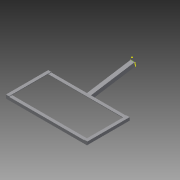
# Autodesk Inventor part: Prow rev2
Saved by Autodesk Inventor 2015 (Build 190159000, 159)
## iProperties
Created: 2016-02-01
Part Number: Prow rev2
Material: Generic
Document SubType Name: Modeling
Designer: sethbattis
Density: 1 g/cm^3
Appearance: Default
Author: sethbattis
Autodesk Inventor part; units mm, degrees
ref_plane "YZ Plane" through (0, 0, 0) normal (1, 0, 0) x (0, 1, 0)
ref_plane "XZ Plane" through (0, 0, 0) normal (0, 1, 0) x (-1, 0, 0)
ref_plane "XY Plane" through (0, 0, 0) normal (0, 0, 1) x (1, 0, 0)
sketch "Sketch1" plane through (0, 0, 0) normal (1, 0, 0) x (0, 1, 0)
  line L0 (-3.175, 114.3) -> (0, 114.3)
  line L1 (0, 114.3) -> (0, 133.35)
  line L2 (0, 133.35) -> (-19.05, 133.35)
  line L3 (-19.05, 133.35) -> (-19.05, 130.175)
  line L4 (-19.05, 130.175) -> (-3.175, 130.175)
  line L5 (-3.175, 130.175) -> (-3.175, 114.3)
  line L6 (0, -114.3) -> (0, -133.35)
  line L7 (0, -133.35) -> (-19.05, -133.35)
  line L8 (-19.05, -133.35) -> (-19.05, -130.175)
  line L9 (-19.05, -130.175) -> (-3.175, -130.175)
  line L10 (-3.175, -130.175) -> (-3.175, -114.3)
  line L11 (-3.175, -114.3) -> (0, -114.3)
  line L12 (-25.4768, 0) -> (19.5105, 0) construction
  line L13 (0, -349.8749) -> (0, 213.8875) construction
  point P0 (0, 0)
  dimension "d0" = 19.05
  dimension "d1" = 19.05
  dimension "d3" = 266.7
  dimension "d4" = 3.175
  constraints: 24 end point, 9 perpendicular, 5 equal length, 2 point on line, 1 collinear, 1 horizontal, 1 vertical, 1 other
  measures "d0" distance of L1.end L2.end
  measures "d1" distance of L0.end L1.end
  measures "d3" distance between parallel lines of L7 L2
  measures "d4" distance of L0.start L0.end
extrude "Extrusion1" add sketch "Sketch1" along normal mid plane 508
sketch "Sketch3" plane through (0, 0, 0) normal (1, 0, 0) x (0, 1, 0)
  line L0 (-25.0873, -137.3234) -> (18.6205, -413.2836)
  line L1 (0, -323.2049) -> (0, 53.8675) projected
  line L2 (-25.0873, -137.3234) -> (0, -133.35)
  line L3 (0, -133.35) -> (43.7078, -409.3101)
  line L4 (43.7078, -409.3101) -> (18.6205, -413.2836)
  point P0 (0, 0)
  dimension "d7" = 9
  dimension "d8" = 279.4
  dimension "d10" = 25.4
  constraints: 8 end point, 3 perpendicular
  measures "d7" angle of L1 L0
  measures "d8" distance of L2.end L3.end
  measures "d10" distance of L2.end L0.start
extrude "Extrusion2" add sketch "Sketch3" along normal mid plane 25.4
sketch "Sketch4" plane through (-254, -19.05, 133.35) normal (0, 0, 1) x (1, 0, 0)
  line L0 (241.3, 19.05) -> (0, 19.05) projected
  line L1 (15.875, 19.05) -> (15.875, 22.225)
  line L2 (15.875, 22.225) -> (-3.175, 22.225)
  line L3 (-3.175, 22.225) -> (-3.175, 3.175)
  line L4 (-3.175, 3.175) -> (0, 3.175)
  line L5 (0, 3.175) -> (0, 19.05)
  line L6 (0, 19.05) -> (15.875, 19.05)
  line L7 (492.028, 19.05) -> (492.028, 22.225)
  line L8 (492.028, 22.225) -> (511.078, 22.225)
  line L9 (511.078, 22.225) -> (511.078, 3.175)
  line L10 (511.078, 3.175) -> (507.903, 3.175)
  line L11 (507.903, 3.175) -> (507.903, 19.05)
  line L12 (507.903, 19.05) -> (492.028, 19.05)
  line L13 (508, 19.05) -> (266.7, 19.05) projected
  line L14 (0, 19.05) -> (508, 19.05) projected
  point P0 (254, 19.05)
  dimension "d13" = 19.05
  dimension "d15" = 3.175
  constraints: 24 end point, 8 perpendicular, 6 equal length, 3 collinear, 2 vertical, 1 point on line
  measures "d13" distance of L7.end L8.end
  measures "d15" distance of L7.start L7.end
extrude "Extrusion3" add sketch "Sketch4" against normal up to surface (266.7 mm away)
sketch "Sketch5" plane through (12.7, 43.7078, -409.3101) normal (0, 0.1564345, -0.9876883) x (-1, 0, 0)
  line L0 (25.4, 0) -> (25.4, -25.4) projected
  line L1 (0, -25.4) -> (0, 0) projected
  line L2 (13.3974, 0) -> (13.3974, -25.4)
  point P0 (12.7, 20.8605)
  constraints: 2 end point, 1 vertical
body "Solid1"
